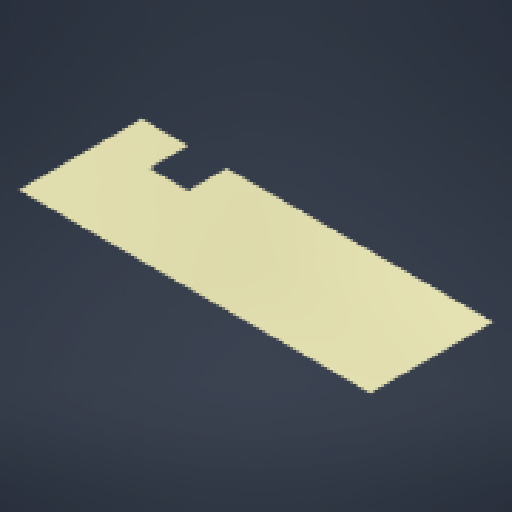
# Autodesk Inventor part: Floor, Floor
Saved by Autodesk Inventor 2026 (Build 300175000, 175)
## iProperties
Created: 2025-11-03
Part Number: Floor, Floor
Material: Polypropylene
Document SubType Name: Sheet Metal
Designer: Brandon Portillo
Density: 0.899 g/cm^3
Sheet Metal Rule: Default
Appearance: Smooth - Ash
Author: Brandon Portillo
Autodesk Inventor part; units mm, degrees
ref_plane "YZ Plane" through (0, 0, 0) normal (1, 0, 0) x (0, 1, 0)
ref_plane "XZ Plane" through (0, 0, 0) normal (0, 1, 0) x (-1, 0, 0)
ref_plane "XY Plane" through (0, 0, 0) normal (0, 0, 1) x (1, 0, 0)
sketch "Sketch1" plane through (0, 0, 0) normal (0, 1, 0) x (-1, 0, 0)
  line L0 (0, 0) -> (-10000, 0)
  line L1 (-10000, 0) -> (-10000, -3500)
  line L2 (-10000, -3500) -> (0, -3500)
  line L3 (0, -3500) -> (0, 0)
  dimension "d0" = 10000
  dimension "d1" = 3500
  measures "d0" distance of L2.end L1.end
  measures "d1" distance of L1.end L0.end
extrude "Plate1" add sketch "Sketch1" along normal blind 2
sketch "Sketch2" plane through (0, 0, 0) normal (0, -1, 0) x (1, 0, 0)
  line L0 (2420, 112.7521) -> (2420, -3617.2479) projected
  line L1 (900, -3726) -> (900, 226) projected
  line L2 (10000, -3500) -> (0, -3500) projected
  line L3 (2420, -3500) -> (1320, -3500)
  line L4 (1320, -3500) -> (1320, -2280)
  line L5 (1320, -2280) -> (2420, -2280)
  line L6 (2420, -2280) -> (2420, -3500)
  line L7 (1353.8656, -2345.1271) -> (1353.8656, -2281.1191) projected
  point P0 (0, 0)
  point P1 (2420, -2280)
  dimension "d3" = 1100
  dimension "d4" = 1220
  constraints: 8 end point, 2 parallel, 2 point on line, 1 horizontal, 1 perpendicular
  measures "d3" distance of L4.end L5.end
  measures "d4" distance of L3.end L4.end
extrude "Cut1" cut sketch "Sketch2" against normal blind 2
equation "\"d5\" = Thickness"
equation "\"d2\" = Thickness"
equation "\"BendRadius\" = Thickness"
equation "\"BendReliefWidth\" = Thickness"
equation "\"BendReliefDepth\" = 0.5 * Thickness"
equation "\"CornerReliefSize\" = 4 * Thickness"
equation "\"MinimumRemnant\" = 2 * Thickness"
equation "\"TransitionRadius\" = BendRadius"
equation "\"JacobiRadiusSize\" = BendRadius"
equation "\"GapSize\" = Thickness"
equation "\"Thickness\" = 2"
body "Solid1"
